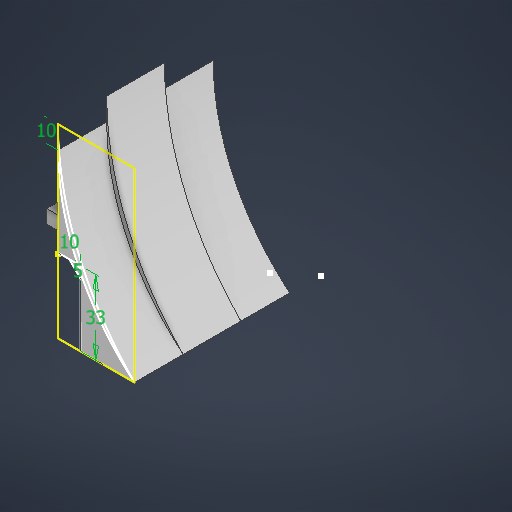
# Autodesk Inventor part: Ramp
Saved by Autodesk Inventor 2026.1 (Build 301233000, 233)
## iProperties
Created: 2026-05-18
Part Number: Ramp
Material: Generic
Document SubType Name: Modeling
Designer: 25adoh
Density: 1 g/cm^3
Appearance: Default
Author: 25adoh
Autodesk Inventor part; units mm, degrees
ref_plane "YZ Plane" through (0, 0, 0) normal (1, 0, 0) x (0, 1, 0)
ref_plane "XZ Plane" through (0, 0, 0) normal (0, 1, 0) x (-1, 0, 0)
ref_plane "XY Plane" through (0, 0, 0) normal (0, 0, 1) x (1, 0, 0)
sketch "Sketch1" plane through (0, 0, 0) normal (1, 0, 0) x (0, 1, 0)
  line L0 (0, -34.5) -> (0, 34.5)
  line L1 (0, 34.5) -> (10, 34.5)
  line L2 (10, 34.5) -> (10, 29.5)
  line L3 (10, 29.5) -> (0, 29.5)
  line L4 (0, 29.5) -> (0, 34.5)
  line L5 (0, 29.5) -> (4, 29.5)
  line L6 (4, 29.5) -> (4, 17.85)
  line L7 (4, 17.85) -> (0, 17.85)
  line L8 (0, 17.85) -> (0, 29.5)
  line L9 (0, 17.85) -> (10, 17.85)
  line L10 (10, 17.85) -> (10, 12.85)
  line L11 (10, 12.85) -> (0, 12.85)
  line L12 (0, 12.85) -> (0, 17.85)
  line L13 (10, 29.5) -> (4, 29.5)
  line L14 (4, 29.5) -> (4, 17.85)
  line L15 (4, 17.85) -> (10, 17.85)
  line L16 (10, 17.85) -> (10, 29.5)
  line L17 (0, -12.85) -> (10, -12.85)
  line L18 (10, -12.85) -> (10, -17.85)
  line L19 (10, -17.85) -> (0, -17.85)
  line L20 (0, -17.85) -> (0, -12.85)
  line L21 (0, -17.85) -> (4, -17.85)
  line L22 (4, -17.85) -> (4, -29.5)
  line L23 (4, -29.5) -> (0, -29.5)
  line L24 (0, -29.5) -> (0, -17.85)
  line L25 (0, -29.5) -> (10, -29.5)
  line L26 (10, -29.5) -> (10, -34.5)
  line L27 (10, -34.5) -> (0, -34.5)
  line L28 (0, -34.5) -> (0, -29.5)
  line L29 (10, -17.85) -> (4, -17.85)
  line L30 (4, -17.85) -> (4, -29.5)
  line L31 (4, -29.5) -> (10, -29.5)
  line L32 (10, -29.5) -> (10, -17.85)
  line L33 (0, 34.5) -> (50, 34.5)
  line L34 (50, 34.5) -> (50, -34.5)
  line L35 (50, -34.5) -> (0, -34.5)
  line L36 (0, -34.5) -> (0, 34.5)
  line L37 (0, 12.85) -> (50, 12.85)
  line L38 (50, 12.85) -> (50, -12.85)
  line L39 (50, -12.85) -> (0, -12.85)
  line L40 (0, -12.85) -> (0, 12.85)
  line L41 (0, -34.5) -> (-32.5, -34.5)
  line L42 (-32.5, -34.5) -> (-32.5, 34.5)
  line L43 (-32.5, 34.5) -> (0, 34.5)
  line L44 (0, 34.5) -> (0, -34.5)
  line L45 (0, 12.85) -> (-32.5, 12.85)
  line L46 (-32.5, 12.85) -> (-32.5, -12.85)
  line L47 (-32.5, -12.85) -> (0, -12.85)
  line L48 (0, -12.85) -> (0, 12.85)
  point P0 (0, 0)
  dimension "d0" = 69
  dimension "d1" = 10
  dimension "d2" = 5
  dimension "d3" = 4
  dimension "d4" = 11.65
  dimension "d5" = 5
  dimension "d6" = 10
  dimension "d7" = 5
  dimension "d8" = 4
  dimension "d9" = 11.65
  dimension "d10" = 5
  dimension "d11" = 50
  dimension "d14" = 32.5
  constraints: 98 end point, 24 parallel, 12 horizontal, 12 perpendicular, 2 point on line, 1 midpoint, 1 vertical
  measures "d0" distance of L0.start L0.end
  measures "d1" distance of L2.end L3.end
  measures "d2" distance of L1.end L2.end
  measures "d3" distance of L6.end L7.end
  measures "d4" distance of L5.end L6.end
  measures "d5" distance of L9.end L10.end
  measures "d6" distance of L29.start L21.start
  measures "d7" distance of L18.start L29.start
  measures "d8" distance of L22.end L23.end
  measures "d9" distance of L21.end L22.end
  measures "d10" distance of L25.end L27.start
  measures "d11" distance of L34.end L35.end
  measures "d14" distance of L42.end L43.end
extrude "Extrusion1" add sketch "Sketch1" along normal blind 34
extrude "Extrusion2" add sketch "Sketch1" against normal blind 10 contours L22 L19 L32 L25 | L6 L3 L16 L9
sketch "Sketch4" plane through (0, -32.5, 34.5) normal (0, 0, 1) x (1, 0, 0)
  line L0 (0, 82.5) -> (0, 0) projected
  line L1 (0, 0) -> (34, 0) projected
  line L2 (34, 82.5) -> (34, 0) projected
  line L3 (0, 82.5) -> (34, 82.5) projected
  line L4 (0, 0) -> (34, 0)
  line L5 (34, 0) -> (34, 82.5)
  line L6 (34, 82.5) -> (0, 82.5)
  line L7 (0, 82.5) -> (0, 0)
  line L8 (0, 0) -> (10, 0)
  line L9 (10, 0) -> (10, 33)
  line L10 (10, 33) -> (0, 33)
  line L11 (0, 33) -> (0, 0)
  line L12 (0, 82.5) -> (0, 72.5)
  arc A0 (0, 72.5) -> (34, 0) centre (94.2978, 72.5) ccw
  arc A1 (0, 82.5) -> (34, 0) centre (117.0919, 82.5) ccw
  line L13 (10, 33) -> (10, 28)
  line L14 (10, 28) -> (5, 33)
  point P0 (0, 32.5)
  point P1 (8.6717, 33)
  point P2 (10, 30.2394)
  dimension "d28" = 10
  dimension "d29" = 33
  dimension "d30" = 10
  dimension "d43" = 5
  constraints: 22 end point, 4 parallel, 4 point on circle, 2 centre point, 2 horizontal, 2 perpendicular, 2 point on line, 2 tangent, 1 midpoint
  measures "d28" distance of L10.end L9.end
  measures "d29" distance of L9.end L8.end
  measures "d30" distance of L6.end L12.end
  measures "d43" distance of L9.end L13.end
extrude "Extrusion6" cut sketch "Sketch4" against normal up to surface (69 mm away) contours A1 A0 L9 L10 L0 | L3 L2 A1 | L10 L9 A0
extrude "Extrusion7" add sketch "Sketch1" along normal blind 34 contours L42 L45 L0 L47 | L0 L11 L37 L34 L39 L17
sketch "Sketch5" plane through (0, 40, 12.85) normal (0, 0, 1) x (1, 0, 0)
  arc A0 (0, 0) -> (34, -72.5) centre (94.2978, 0) ccw projected
  line L0 (34, 10) -> (34, -72.5) projected
  line L1 (0, 10) -> (34, 10) projected
  line L2 (0, 10) -> (0, 0) projected
  arc A1 (0, 10) -> (34, -72.5) centre (117.0919, 10) ccw
  point P0 (0, -40)
  constraints: 2 point on circle, 1 centre point, 1 tangent
extrude "Extrusion8" cut sketch "Sketch5" against normal up to surface (25.7 mm away) contours A1 L1 L0
extrude "Extrusion9" cut sketch "Sketch4" against normal blind 15 contours L10 L14 L9 L1 L0
sketch "Sketch6" plane through (0, -32.5, -34.5) normal (0, 0, -1) x (-1, 0, 0)
  line L0 (-10, 0) -> (0, 0) projected
  line L1 (0, 0) -> (-10, 0)
  line L2 (-10, 0) -> (-10, 33)
  line L3 (-10, 33) -> (0, 33)
  line L4 (0, 33) -> (0, 0)
  line L5 (-5, 33) -> (-10, 28) projected
  line L6 (-10, 28) -> (-5, 33)
  point P0 (0, 32.5)
  dimension "d39" = 10
  dimension "d40" = 33
  constraints: 10 end point, 3 equal length, 1 horizontal, 1 perpendicular, 1 point on line
  measures "d39" distance of L2.end L3.end
  measures "d40" distance of L1.end L2.end
extrude "Extrusion10" cut sketch "Sketch6" against normal blind 15 contours L2 L5 L3 L4 L0
body "Solid1"
